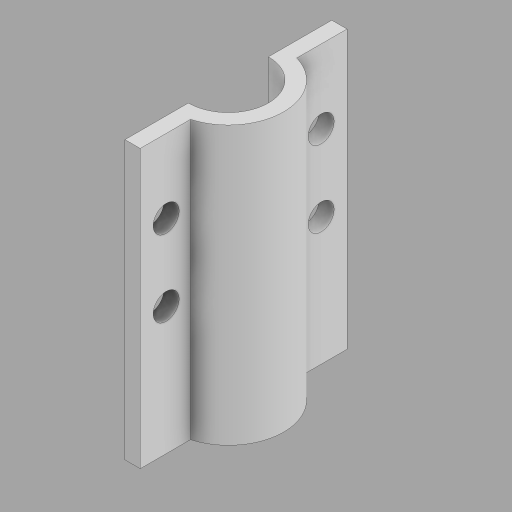
# Autodesk Inventor part: pen고정부
Saved by Autodesk Inventor 2023.1 (Build 271208000, 208)
## iProperties
Created: 2022-10-29
Part Number: pen고정부
Material: 일반
Document SubType Name: Modeling
Designer: 박동준
Density: 1 g/cm^3
Appearance: 기본값
Author: 박동준
Autodesk Inventor part; units mm, degrees
ref_plane "YZ Plane" through (0, 0, 0) normal (1, 0, 0) x (0, 1, 0)
ref_plane "XZ Plane" through (0, 0, 0) normal (0, 1, 0) x (-1, 0, 0)
ref_plane "XY Plane" through (0, 0, 0) normal (0, 0, 1) x (1, 0, 0)
sketch "스케치1" plane through (0, 0, 0) normal (0, 1, 0) x (-1, 0, 0)
  arc A0 (0, 5.25) -> (0, -5.25) centre (0, 0) ccw
  line L0 (0, 0) -> (0, 5.25) construction
  line L1 (0, 0) -> (5.25, 0) construction
  line L2 (0, 0) -> (0, -5.25) construction
  arc A1 (-2, 6.9687) -> (-2, -6.9687) centre (0, 0) ccw
  line L3 (0, 0) -> (0, -9) construction
  line L4 (0, 0) -> (0, 9) construction
  line L5 (0, 5.25) -> (0, 13.57)
  line L6 (0, 13.57) -> (-2, 13.57)
  line L7 (-2, 13.57) -> (-2, 6.9687)
  line L8 (0, -5.25) -> (0, -13.57)
  line L9 (0, -13.57) -> (-2, -13.57)
  line L10 (-2, -13.57) -> (-2, -6.9687)
  point P0 (-1, -13.57)
  point P1 (-1, 13.57)
  dimension "d46" = 5.25
  dimension "d47" = 90
  dimension "d48" = 180
  dimension "d49" = 7.25
  dimension "d50" = 180
  dimension "d51" = 13.57
  dimension "d52" = 13.57
  dimension "d53" = 2
  dimension "d54" = 2
  constraints: 22 end point, 5 perpendicular, 4 point on circle, 2 centre point, 2 coincident, 2 midpoint, 2 vertical, 1 horizontal
  measures "d46" radius of A0
  measures "d47" angle of L1 L0
  measures "d48" angle of L2 L0
  measures "d49" radius of A1
  measures "d50" angle of L4 L3
  measures "d51" vertical distance of point (0, 0) point (-1, -13.57)
  measures "d52" vertical distance of point (0, 0) point (-1, 13.57)
  measures "d53" distance of L5.end L6.end
  measures "d54" distance of L8.end L9.end
extrude "돌출1" add sketch "스케치1" along normal blind 36.4
sketch "스케치2" plane through (2, 0, 13.57) normal (1, 0, 0) x (0, 0, -1)
  line L0 (0, 0) -> (6.6013, 0) projected
  line L1 (6.6013, 0) -> (6.6013, 36.4) projected
  line L2 (0, 36.4) -> (6.6013, 36.4) projected
  line L3 (0, 0) -> (0, 36.4) projected
  circle A0 centre (3.4, 26.75) radius 1.7
  circle A1 centre (3.4, 16.75) radius 1.7
  point P0 (13.57, 0)
  point P1 (3.3007, 36.4)
  dimension "d57" = 3.4
  dimension "d58" = 3.4
  dimension "d60" = 26.75
  dimension "d61" = 16.75
  dimension "d64" = 3.4
  constraints: 2 centre point, 1 midpoint, 1 vertical alignment
  measures "d57" diameter of A0
  measures "d58" diameter of A1
  measures "d60" distance from line of L0 A0.centre
  measures "d61" distance from line of L0 A1.centre
  measures "d64" distance from line of A0.centre L3
extrude "돌출2" cut sketch "스케치2" against normal through all contours A0 | A1
mirror "미러2" about plane through (0, 0, 0) normal (0, 0, 1) of "돌출2"
